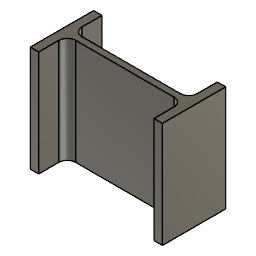
H-125×60×6×8 (Autodesk Fusion 360 design; units mm, degrees)
Autodesk Fusion 360 part; units mm, degrees
sketch "スケッチ1" plane through (0, 0, 0) normal (0, 0, 1) x (1, 0, 0)
  line L0 (0, 30) -> (0, -30)
  line L1 (8, 11) -> (8, 30)
  line L2 (117, 30) -> (117, 11)
  line L3 (125, -30) -> (125, 30)
  line L4 (109, 3) -> (16, 3)
  line L5 (16, -3) -> (109, -3)
  line L6 (0, -30) -> (8, -30)
  line L7 (8, -30) -> (8, -11)
  line L8 (117, -30) -> (125, -30)
  line L9 (117, -11) -> (117, -30)
  line L10 (8, 30) -> (0, 30)
  line L11 (125, 30) -> (117, 30)
  arc A0 (8, 11) -> (16, 3) centre (16, 11) ccw
  arc A1 (16, -3) -> (8, -11) centre (16, -11) ccw
  arc A2 (117, -11) -> (109, -3) centre (109, -11) ccw
  arc A3 (109, 3) -> (117, 11) centre (109, 11) ccw
extrude "押し出し1" add sketch "スケッチ1" along normal blind 100
